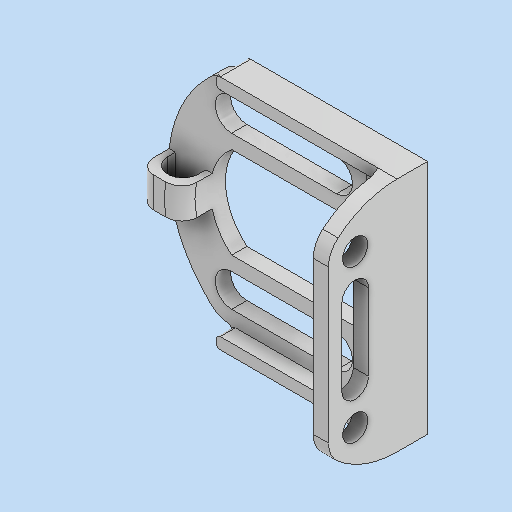
# Autodesk Inventor part: X-Gantry Enstop Mount
Saved by Autodesk Inventor 2023.2 (Build 272271000, 271)
## iProperties
Created: 2024-02-13
Part Number: X-Gantry Enstop Mount
Material: Generisch
Document SubType Name: Modeling
Designer: Nils Bade
Density: 1 g/cm^3
Appearance: Resin-3D-Druck
Auf Bestellliste: True
Author: Nils Bade
Autodesk Inventor part; units mm, degrees
ref_plane "YZ Plane" through (0, 0, 0) normal (1, 0, 0) x (0, 1, 0)
ref_plane "XZ Plane" through (0, 0, 0) normal (0, 1, 0) x (-1, 0, 0)
ref_plane "XY Plane" through (0, 0, 0) normal (0, 0, 1) x (1, 0, 0)
sketch "S-Schiene" plane through (0, 0, 0) normal (0, 0, 1) x (1, 0, 0)
  line L0 (-30.84, 0) -> (5.14, 0) projected
  line L1 (0, -9.1) -> (0, 19.6) projected
  circle A0 centre (-8.5116, 10) radius 2.15 construction
  circle A1 centre (-8.5116, 10) radius 3.5 construction
  line L2 (-4, 10) -> (-21.7, 10) construction
  line L3 (-4, 12.15) -> (-21.7, 12.15)
  line L4 (-21.7, 7.85) -> (-4, 7.85)
  arc A2 (-4, 7.85) -> (-4, 12.15) centre (-4, 10) ccw
  arc A3 (-21.7, 12.15) -> (-21.7, 7.85) centre (-21.7, 10) ccw
  line L5 (-4, 10) -> (-21.7, 10) construction
  line L6 (0, 14) -> (-21.7, 14)
  line L7 (-21.7, 6) -> (0, 6)
  arc A4 (-4, 6) -> (-4, 14) centre (-4, 10) ccw construction
  arc A5 (-21.7, 14) -> (-21.7, 6) centre (-21.7, 10) ccw
  circle A6 centre (-7.7662, 0) radius 5 construction
  line L8 (-21.7, 10) -> (-8, 10) construction
  line L9 (-21.7, 7.8491) -> (-8, 7.8491)
  line L10 (-8, 12.1509) -> (-21.7, 12.1509)
  arc A7 (-21.7, 12.1509) -> (-21.7, 7.8491) centre (-21.7, 10) ccw
  arc A8 (-8, 7.8491) -> (-8, 12.1509) centre (-8, 10) ccw
  line L11 (0, 14) -> (-21.7, 14)
  line L12 (-21.7, 14) -> (-21.7, 15.5)
  line L13 (-21.7, 15.5) -> (0, 15.5)
  line L14 (0, 15.5) -> (0, 14)
  point P0 (-12.85, 10)
  point P1 (-12.85, 10)
  point P2 (0, 10)
  point P3 (-23.85, 10)
  point P4 (-1.85, 10)
  point P5 (0, 0)
  point P6 (-14.85, 10)
  point P7 (-7.9383, 12.15)
  point P8 (-7.9383, 7.85)
  point P9 (0, 15.5)
  dimension "d1" = 4.3
  dimension "d2" = 7
  dimension "d3" = 10
  dimension "d4" = 4.3
  dimension "d5" = 8
  dimension "d6" = 22
  dimension "d10" = 10
  dimension "d24" = 4
  dimension "d45" = 1.5
  constraints: 32 end point, 15 point on circle, 12 tangent, 9 centre point, 8 point on line, 6 equal length, 3 midpoint, 2 perpendicular, 1 coincident, 1 horizontal
  measures "d1" diameter of A0
  measures "d2" diameter of A1
  measures "d3" distance from line of A0.centre L0
  measures "d4" diameter of A3
  measures "d5" diameter of A5
  measures "d6" distance of point (-23.85, 10) point (-1.85, 10)
  measures "d10" diameter of A6
  measures "d24" distance of L2.start L8.end
  measures "d45" distance between parallel lines of L11 L13
extrude "Ex-Schiene" add sketch "S-Schiene" along normal blind 2 contours L7 A5 L6 L1 | A2 L4 A8 L3
extrude "Ex-Biegesteifigkeit" add sketch "S-Schiene" along normal blind 4 contours L6 L12 L13 L1
sketch "S-Front" plane through (0, 0, 0) normal (1, 0, 0) x (0, 1, 0)
  circle A0 centre (10, 9.5) radius 1.65
  circle A1 centre (10, 9.5) radius 3
  line L0 (6, 2) -> (14, 2) construction
  line L1 (0, 9.5) -> (5.0327, 9.5) construction
  line L2 (0, 7.75) -> (5.0327, 7.75)
  line L3 (5.0327, 11.25) -> (0, 11.25)
  arc A2 (0, 11.25) -> (0, 7.75) centre (0, 9.5) ccw construction
  arc A3 (5.0327, 7.75) -> (5.0327, 11.25) centre (5.0327, 9.5) ccw
  line L4 (0, 15.6) -> (0, -2.6) projected
  line L5 (0, 9.5) -> (10, 9.5) construction
  line L6 (0, 6) -> (10, 6) construction
  line L7 (10, 13) -> (0, 13)
  arc A4 (0, 13) -> (0, 6) centre (0, 9.5) ccw construction
  arc A5 (10, 6) -> (10, 13) centre (10, 9.5) ccw
  line L8 (14, 0) -> (14, 2) projected
  line L9 (6, 0) -> (14, 0) projected
  line L10 (6, 0) -> (6, 2) projected
  line L11 (6, 0) -> (0, 0)
  line L12 (14, 2) -> (6, 2) projected
  line L13 (15.5, 0) -> (15.5, 4) projected
  arc A6 (15.5, 4) -> (12.6825, 11.7482) centre (3.4375, 4) ccw
  line L14 (6, 0) -> (15.5, 0) projected
  line L15 (15.5, 0) -> (15.5, 4) projected
  line L16 (14, 4) -> (15.5, 4) projected
  line L17 (14, 2) -> (14, 4) projected
  line L18 (6, 2) -> (14, 2) projected
  line L19 (6, 0) -> (6, 2) projected
  point P0 (2.5163, 9.5)
  point P1 (5, 9.5)
  point P2 (0, 13)
  dimension "d11" = 3.3
  dimension "d13" = 6
  dimension "d15" = 3.5
  dimension "d16" = 7
  dimension "d23" = 9.5
  constraints: 18 end point, 11 point on circle, 10 tangent, 7 centre point, 2 coincident, 2 midpoint, 2 parallel, 1 perpendicular, 1 point on line
  measures "d11" diameter of A0
  measures "d13" diameter of A1
  measures "d15" diameter of A3
  measures "d16" diameter of A5
  measures "d23" distance from line of L9 A0.centre
extrude "Ex-Front" add sketch "S-Front" along normal blind 2 contours A1 | L2 A3 L3 L4 L7 A5 A6 L16 L17 L12 L10 L11 | L10 L12 L8 L9 | L8 L17 L16 L13 L14
fillet "Rundung-4mm" radius 4 2 edges at (0, 6, 1) (0, 10, 2)
extrude "Ex-SchraubenkopfEinlasss" [suppressed]
mirror "Spiegeln2" about plane through (0, 0, 0) normal (0, 1, 0)
ref_plane "E-Slide1" through (-21.7, 10, 0) normal (0, -1, 0) x (1, 0, 0)
ref_plane "E-slide2" through (-21.7, -10, 0) normal (0, -1, 0) x (1, 0, 0)
sketch "S-Extension" plane through (0, 0, 0) normal (0, 0, 1) x (1, 0, 0)
  arc A0 (-21.7, 14) -> (-21.7, 6) centre (-21.7, 10) ccw projected
  arc A1 (-21.7, -6) -> (-21.7, -14) centre (-21.7, -10) ccw projected
  arc A2 (-21.7, -6) -> (-21.7, -14) centre (-21.7, -10) ccw projected
  arc A3 (-21.7, 6) -> (-21.7, -6) centre (-16.7051, 0) ccw
  arc A4 (-21.7, 14) -> (-21.7, 6) centre (-21.7, 10) ccw projected
  arc A5 (-24.4064, 12.9454) -> (-24.4456, -12.9089) centre (-12.2613, -0.0002) ccw
  line L0 (-24.2516, 2) -> (-29.8991, 2)
  line L1 (-36.0381, 0) -> (6.0063, 0) construction
  line L2 (-29.8991, -2) -> (-24.2516, -2)
  point P0 (0, 0)
  point P1 (-24.4843, 12.8718)
  point P2 (-24.4456, -12.9089)
  dimension "d34" = 2
  dimension "d36" = 2
  constraints: 10 point on circle, 4 end point, 2 centre point, 2 horizontal, 1 tangent
  measures "d34" distance between parallel lines of L1 L0
  measures "d36" distance between parallel lines of L2 L1
extrude "Ex-Extension1" add sketch "S-Extension" along normal blind 2
extrude "Ex-Extension2" add sketch "S-Extension" along normal blind 6 contours L0 A3 L2 A5
sketch "Skizze5" plane through (-29.8991, -2, 2) normal (0, -1, 0) x (1, 0, 0)
  line L0 (5.6475, 0) -> (0, 0) projected
  line L1 (5.6475, 0) -> (5.6475, 4) projected
  line L2 (0, 4) -> (5.6475, 4) projected
  line L3 (0, 0) -> (0, 4) projected
  line L4 (5.4148, 0) -> (0, 0) projected
  line L5 (0.8238, 0) -> (4.8238, 0)
  line L6 (4.8238, 0) -> (4.8238, 3)
  line L7 (4.8238, 3) -> (0.8238, 3)
  line L8 (0.8238, 3) -> (0.8238, 0)
  line L9 (0, 4) -> (5.6475, 4) construction
  line L10 (2.8238, 4) -> (2.8238, 0) construction
  point P0 (29.8991, -2)
  point P1 (2.8238, 3)
  point P2 (0.8238, 0)
  point P3 (4.8238, 0)
  dimension "d40" = 4
  dimension "d41" = 3
  constraints: 10 end point, 3 midpoint, 2 parallel, 2 point on line, 1 horizontal, 1 perpendicular
  measures "d40" distance between parallel lines of L6 L8
  measures "d41" distance between parallel lines of L0 L7
extrude "Ex-Extension3" cut sketch "Skizze5" against normal up to surface (4 mm away) contours L0 L8 L7 L6
fillet "Rundung-2mm" radius 2 4 edges at (-25.0753, 0, 5) (-29.0753, 0, 5) (-24.5121, 0, 6) (-30.0121, 0, 6)
fillet "Rundung-0.5mm" radius 0.5 6 edges at (-21.7, 14, 1) (-21.7, 15.5, 2) (-21.7, 14, 3) (-21.7, -14, 3) (-21.7, -14, 1) (-21.7, -15.5, 2)
equation "\"d36\" = d34"
